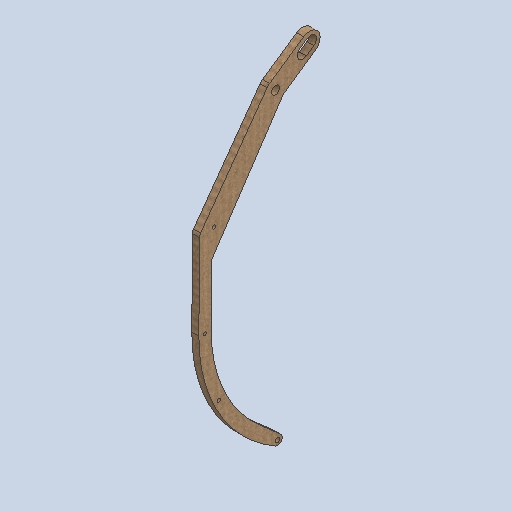
# Autodesk Inventor part: hand-grab-v1-POM-arm
Saved by Autodesk Inventor 2025.1 (Build 291241000, 241)
## iProperties
Created: 2024-10-07
Part Number: hand-grab-v1-POM-arm
Material: MDF 中密度繊維ボード
Document SubType Name: Modeling
Designer: haruy
Density: 0.8 g/cm^3
Appearance: ダンボール - 段ボール紙
Author: haruy
Autodesk Inventor part; units mm, degrees
ref_plane "YZ Plane" through (0, 0, 0) normal (1, 0, 0) x (0, 1, 0)
ref_plane "XZ Plane" through (0, 0, 0) normal (0, 1, 0) x (-1, 0, 0)
ref_plane "XY Plane" through (0, 0, 0) normal (0, 0, 1) x (1, 0, 0)
derived "hand-grab-v1-Sketch-Base.ipt"
sketch "スケッチ1" plane through (400, 0, 0) normal (1, 0, 0) x (0, 1, 0)
  circle A0 centre (0, 0) radius 120
  circle A1 centre (-109.5522, 63.25) radius 6.5 construction
  line L0 (0, 0) -> (-109.5522, 63.25) construction
  line L1 (0, 0) -> (0, 120)
  line L2 (246.0862, 200) -> (-251.4603, 200)
  circle A2 centre (145, 60) radius 254.573 construction
  circle A3 centre (-67.6203, 200) radius 6.5
  line L3 (0, 0) -> (-120, 0)
  line L4 (249, 9.15) -> (187, 9.15)
  line L5 (187, 9.15) -> (187, -9.15)
  line L6 (187, -9.15) -> (249, -9.15)
  line L7 (249, -9.15) -> (249, 9.15)
  line L8 (187, 5.15) -> (179, 5.15)
  line L9 (179, 5.15) -> (179, -4.85)
  line L10 (179, -4.85) -> (187, -4.85)
  line L11 (187, -4.85) -> (187, 5.15)
  line L12 (179, 3.15) -> (174, 3.15)
  line L13 (174, 3.15) -> (174, -2.85)
  line L14 (174, -2.85) -> (179, -2.85)
  line L15 (179, -2.85) -> (179, 3.15)
  line L16 (174, 2.65) -> (159, 2.65)
  line L17 (159, 2.65) -> (159, -2.35)
  line L18 (159, -2.35) -> (174, -2.35)
  line L19 (174, -2.35) -> (174, 2.65)
  line L20 (187, 34.15) -> (184, 34.15)
  line L21 (184, 34.15) -> (184, -43.5182)
  line L22 (184, -43.5182) -> (187, -43.5182)
  line L23 (187, -43.5182) -> (187, 34.15)
  circle A4 centre (150, 65) radius 4 construction
  circle A5 centre (150, 65) radius 14 construction
  line L24 (187, 34.15) -> (192, 34.15)
  line L25 (192, 34.15) -> (192, 14.15)
  line L26 (192, 14.15) -> (187, 14.15)
  line L27 (187, 14.15) -> (187, 34.15)
  line L28 (184, 34.15) -> (147.5804, 61.8148) construction
  line L29 (151.3533, 68.7641) -> (192, 54.15) construction
  line L30 (192, 54.15) -> (192, 34.15)
  line L31 (239.3868, 130) -> (-239.3868, 130) construction
  circle A6 centre (-109.5522, 63.25) radius 4
  circle A7 centre (150, 65) radius 9
  line L32 (-106.0881, 61.25) -> (-113.0163, 65.25) construction
  circle A8 centre (-109.5522, 63.25) radius 2
  circle A9 centre (150, 65) radius 3.5
  line L33 (170, 36) -> (155, 36) construction
  circle A10 centre (155, 36) radius 5 construction
  circle A11 centre (155, 36) radius 9 construction
  circle A12 centre (-90.698, 156.1969) radius 6.5
  circle A13 centre (170, 36) radius 5 construction
  line L34 (150, 65) -> (170, 36) construction
  circle A14 centre (170, 36) radius 9
  circle A15 centre (150, 65) radius 44.2278
  line L35 (150, 65) -> (155, 36) construction
  line L36 (150, 65) -> (-109.5522, 63.25) construction
  line L37 (-90.698, 156.1969) -> (150, 65) construction
  line L38 (150, 65) -> (157.5146, 21.4152) construction
  circle A16 centre (150, 65) radius 35.2278 construction
  circle A17 centre (155.9855, 30.2844) radius 9 construction
  line L39 (168.0777, 21.2844) -> (136, 21.2844)
  circle A18 centre (150, 65) radius 29.4279 construction
  circle A19 centre (166.7072, 40.7746) radius 5 construction
  circle A20 centre (166.1394, 41.5978) radius 5
  line L40 (150, 65) -> (175.1096, 28.5911) construction
  circle A21 centre (170.5677, 35.1768) radius 5
  line L41 (170.2555, 44.4365) -> (174.6838, 38.0155)
  line L42 (162.0234, 38.7591) -> (166.4517, 32.3381)
  line L43 (177.4089, 41.1096) -> (157.4089, 70.1096)
  line L44 (142.5911, 59.8904) -> (162.5911, 30.8904)
  circle A22 centre (0, 0) radius 130.5
  line L45 (-106.5522, 60.6042) -> (-89.9997, 79.3729)
  line L46 (75, 130) -> (75, 0)
  line L47 (0.8751, 130.4971) -> (75, 130)
  line L48 (0, 120) -> (75, 120)
  line L49 (75, 130) -> (155.2533, 72.3077)
  line L50 (51.286, 120) -> (145.0073, 57.5118)
  circle A23 centre (-55, 113.3438) radius 1.5
  circle A24 centre (0, 125.5028) radius 1.5
  circle A25 centre (75, 117.5) radius 1.5
  line L51 (-55, 118.3438) -> (-55, 0)
  line L52 (175, 3.15) -> (175, -2.85)
  point P0 (183.6584, 45.0807)
  point P1 (161.8695, 55.9751)
  point P2 (-60, 0)
  point P3 (138.2515, 64.0454)
  point P4 (151.7485, 75.9546)
  point P5 (143.5711, 58.4694)
  point P6 (-113.0163, 65.25)
  point P7 (75, 104.1888)
  dimension "d1" = 4
  dimension "d2" = 7
  dimension "d8" = 10
  dimension "d9" = 10
  dimension "d10" = 1
  dimension "d11" = 10
  dimension "d12" = 1
  dimension "d13" = 75
  dimension "d15" = 3
  dimension "d16" = 3
  dimension "d17" = 3
  dimension "d18" = 5
  dimension "d19" = 0
  dimension "d20" = 55
  dimension "d21" = 5
  dimension "d22" = 75
  dimension "d23" = 12.5
  measures "d1" diameter of A8
  measures "d2" diameter of A9
  measures "d8" diameter of A19
  measures "d9" diameter of A20
  measures "d10" distance of A20.centre A19.centre
  measures "d11" diameter of A21
  measures "d12" distance of L34.end A21.centre
  measures "d13" distance between parallel lines of L46 L1
  measures "d15" diameter of A23
  measures "d16" diameter of A24
  measures "d17" diameter of A25
  measures "d18" distance from line of L47 A24.centre
  measures "d19" horizontal distance of point (0, 0) A24.centre
  measures "d20" distance from line of A23.centre L1
  measures "d21" distance of L51.start A23.centre
  measures "d22" distance from line of A25.centre L1
  measures "d23" distance of L46.start A25.centre
sketch "スケッチ2" plane through (0, 400, 0) normal (0, 1, 0) x (-1, 0, 0)
  circle A0 centre (0, 0) radius 120
  line L0 (0, 0) -> (-331.4625, 0)
  line L1 (67.5, -116.9134) -> (-135, 0)
  circle A1 centre (0, 0) radius 5
  line L2 (0, 0) -> (67.5, 116.9134)
  line L3 (0, 0) -> (67.5, -116.9134)
  line L4 (0, 0) -> (-135, 0)
  line L5 (17.0359, 37.507) -> (12.0359, 28.8468)
  line L6 (12.0359, 28.8468) -> (15.5, 26.8468)
  line L7 (15.5, 26.8468) -> (20.5, 35.507)
  line L8 (20.5, 35.507) -> (17.0359, 37.507)
  line L9 (20.5, 35.507) -> (15.5, 26.8468)
  line L10 (15.5, 26.8468) -> (18.9641, 24.8468)
  line L11 (18.9641, 24.8468) -> (23.9641, 33.507)
  line L12 (23.9641, 33.507) -> (20.5, 35.507)
  line L13 (14.5359, 33.1769) -> (21.4641, 29.1769)
  circle A2 centre (0, 0) radius 2.65
  line L14 (16.8194, 37.632) -> (10.3194, 26.3737)
  line L15 (10.3194, 26.3737) -> (5.9893, 28.8737)
  line L16 (5.9893, 28.8737) -> (12.4893, 40.132)
  line L17 (12.4893, 40.132) -> (16.8194, 37.632)
  line L18 (28.5107, 30.882) -> (24.1806, 33.382)
  line L19 (22.0107, 19.6237) -> (28.5107, 30.882)
  line L20 (24.1806, 33.382) -> (17.6806, 22.1237)
  line L21 (17.6806, 22.1237) -> (22.0107, 19.6237)
  circle A3 centre (0, 0) radius 28.3207
  line L22 (-41, 9.25) -> (-41, 4.25)
  line L23 (-41, 4.25) -> (-28, 4.25)
  line L24 (-28, 9.25) -> (-41, 9.25)
  line L25 (-28, 4.25) -> (-28, 9.25)
  line L26 (-41, -4.25) -> (-28, -4.25)
  line L27 (-41, -9.25) -> (-41, -4.25)
  line L28 (-28, -9.25) -> (-41, -9.25)
  line L29 (-28, -4.25) -> (-28, -9.25)
  line L30 (12.4893, -40.132) -> (16.8194, -37.632)
  line L31 (16.8194, -37.632) -> (10.3194, -26.3737)
  line L32 (5.9893, -28.8737) -> (12.4893, -40.132)
  line L33 (10.3194, -26.3737) -> (5.9893, -28.8737)
  line L34 (24.1806, -33.382) -> (17.6806, -22.1237)
  line L35 (28.5107, -30.882) -> (24.1806, -33.382)
  line L36 (22.0107, -19.6237) -> (28.5107, -30.882)
  line L37 (17.6806, -22.1237) -> (22.0107, -19.6237)
  line L38 (5.9893, 28.8737) -> (5.373, 27.8064)
  line L39 (22.0107, 19.6237) -> (21.3945, 18.5564)
  line L40 (-28, 9.25) -> (-26.7675, 9.25)
  line L41 (-28, -9.25) -> (-26.7675, -9.25)
  line L42 (5.9893, -28.8737) -> (2.1934, -22.2991)
  line L43 (22.0107, -19.6237) -> (21.3945, -18.5564)
  line L44 (13.6109, 31.5748) -> (3.6109, 14.2543)
  line L45 (3.6109, 14.2543) -> (-1.5853, 17.2543)
  line L46 (-1.5853, 17.2543) -> (8.4147, 34.5748)
  line L47 (8.4147, 34.5748) -> (13.6109, 31.5748)
  circle A4 centre (3.5128, 20.0844) radius 1.5
  circle A5 centre (8.5128, 28.7446) radius 1.5
  circle A6 centre (20.6372, 21.7446) radius 1.5
  circle A7 centre (15.6372, 13.0844) radius 1.5
  circle A8 centre (-29.15, 7) radius 1.5
  circle A9 centre (-19.15, 7) radius 1.5
  circle A10 centre (-19.15, -7) radius 1.5
  circle A11 centre (-29.15, -7) radius 1.5
  circle A12 centre (8.5128, -28.7446) radius 1.5
  circle A13 centre (3.5128, -20.0844) radius 1.5
  circle A14 centre (15.6372, -13.0844) radius 1.5
  circle A15 centre (20.6372, -21.7446) radius 1.5
  line L48 (1.0128, 15.7543) -> (13.6109, 31.5748)
  circle A16 centre (0, 0) radius 34.3835
  line L49 (-8, 47) -> (-188, 47)
  line L50 (-188, 47) -> (-188, 32)
  line L51 (-188, 32) -> (-8, 32)
  line L52 (-8, 32) -> (-8, 47)
ref_plane "作業平面1" through (400, 0, 0) normal (1, 0, 0) x (0, 1, 0)
ref_plane "作業平面2" through (0, 400, 0) normal (0, 1, 0) x (-1, 0, 0)
extrude "押し出し1" add sketch "スケッチ1" along normal blind 6 contours L45 A6 A22 L51 A23 A0 | L51 A23 A22 L48 A0 | A6 | L51 A23 | A23 L51 | L48 L46 A25 A22 | A22 L47 L46 L48 | A22 L46 L50 | L46 A22 L50 | L46 A25 L49 A15 L50 A22 | A25 L46 | L46 A25 | A15 L49 A7 L44 L50 | L50 A7 L43 A14 A20 L44 | L44 A7 L50 | A14 A20 L42 A21 L41 | A7 | A24
fillet "フィレット2" radius 5 3 edges at (403, 75, 130) (403, 51.286, 120) (403, 143.5711, 58.4694)
extrude "押し出し3" cut sketch "スケッチ1" along normal blind 6 contours L51 A23 | A23 L51 | A25 L46 | L46 A25 | A24
sketch "スケッチ4" plane through (406, 0, 120) normal (1, 0, 0) x (0, 0, -1)
  circle A0 centre (6.6562, -55) radius 1.5 projected
  circle A1 centre (-5.5028, 0) radius 1.5 projected
  circle A2 centre (2.5, 75) radius 1.5 projected
  arc A3 (-9.0706, 76.2928) -> (-10.0107, 73.4078) centre (-5.0108, 73.3743) ccw projected
  line L0 (-10.0107, 73.4078) -> (-10.4971, 0.8751) projected
  arc A4 (-10.4971, 0.8751) -> (54.75, -113.0163) centre (120, 0) ccw projected
  arc A5 (54.75, -113.0163) -> (59.3958, -106.5522) centre (56.75, -109.5522) ccw projected
  line L1 (59.3958, -106.5522) -> (40.6271, -89.9997) projected
  arc A6 (0, 0) -> (40.6271, -89.9997) centre (120, 0) ccw projected
  line L2 (0, 0) -> (0, 49.7719) projected
  arc A7 (0.8399, 52.5457) -> (0, 49.7719) centre (5, 49.7719) ccw projected
  line L3 (0.8399, 52.5457) -> (60.9986, 142.7732) projected
  arc A8 (62.32, 144.1155) -> (60.9986, 142.7732) centre (65.1587, 139.9995) ccw projected
  line L4 (62.32, 144.1155) -> (89.1096, 162.5911) projected
  arc A9 (89.1096, 162.5911) -> (78.8904, 177.4089) centre (84, 170) ccw projected
  line L5 (78.8904, 177.4089) -> (49.8904, 157.4089) projected
  arc A10 (49.8904, 157.4089) -> (47.6923, 155.2533) centre (55, 150) ccw projected
  line L6 (47.6923, 155.2533) -> (-9.0706, 76.2928) projected
  circle A11 centre (56.75, -109.5522) radius 2 projected
  circle A12 centre (55, 150) radius 3.5 projected
  arc A13 (75.5635, 170.2555) -> (81.2409, 162.0234) centre (78.4022, 166.1394) ccw projected
  line L7 (75.5635, 170.2555) -> (81.9845, 174.6838) projected
  arc A14 (87.6619, 166.4517) -> (81.9845, 174.6838) centre (84.8232, 170.5677) ccw projected
  line L8 (87.6619, 166.4517) -> (81.2409, 162.0234) projected
